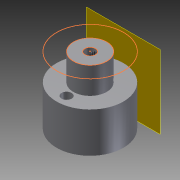
# Autodesk Inventor part: Jig_Bearing_Asm_Housing_Holder
Saved by Autodesk Inventor 2011 SP1 (Build 150282100, 282)
## iProperties
Created: 2011-04-25
Part Number: Jig_Bearing_Asm_Housing_Holder
Document SubType Name: Modeling
Designer: sungwook
Density: 1 g/cm^3
Author: sungwook
Autodesk Inventor part; units mm, degrees
ref_plane "YZ Plane" through (0, 0, 0) normal (1, 0, 0) x (0, 1, 0)
ref_plane "XY Plane" through (0, 0, 0) normal (0, 0, 1) x (1, 0, 0)
sketch "Sketch1" plane through (0, 0, 0) normal (0, 0, 1) x (1, 0, 0)
  circle A0 centre (0, 0) radius 5
  dimension "d0" = 10
  constraints: 1 centre point, 1 coincident
  measures "d0" diameter of A0
extrude "Extrusion1" add sketch "Sketch1" along normal blind 10
sketch "Sketch2" plane through (0, 0, 10) normal (0, 0, 1) x (1, 0, 0)
  circle A0 centre (0, 0) radius 5 projected
  circle A1 centre (0, 0) radius 0.8
  dimension "d3" = 1.6
  constraints: 1 centre point, 1 coincident
  measures "d3" diameter of A1
extrude "Extrusion2" cut sketch "Sketch2" against normal blind 2 contours A1
sketch "Sketch3" plane through (0, 0, 10) normal (0, 0, 1) x (1, 0, 0)
  circle A0 centre (0, 0) radius 0.8 projected
  circle A1 centre (0, 0) radius 5 projected
ref_plane "Work Plane1" through (0, 5, 0) normal (0, 1, 0) x (-1, 0, 0)
sketch "Sketch4" plane through (0, 5, 0) normal (0, 1, 0) x (-1, 0, 0)
  line L0 (-5, 0) -> (-5, 10) projected
  line L1 (5, 0) -> (5, 10) projected
  line L2 (0, -2) -> (0, 12) projected
  line L3 (-5, 10) -> (5, 10) projected
  point P0 (0, 0)
  point P1 (0, 9)
  dimension "d8" = 1
  constraints: 1 point on line
  measures "d8" distance from line of point (0, 9) L3
hole "Hole1" at (0, 5, 9) direction (0, -1, 0) diameter 1.181 depth 5 thread size "0-80 UNF" class "2B" standard "ANSI Unified Screw Threads"
sketch "Sketch5" plane through (0, 0, 10) normal (0, 0, 1) x (1, 0, 0)
  circle A0 centre (0, 0) radius 5 projected
  circle A1 centre (0, 0) radius 2.5
  circle A2 centre (0, 0) radius 5
  dimension "d16" = 5
  constraints: 2 centre point, 2 coincident, 1 concentric
  measures "d16" diameter of A1
extrude "Extrusion3" cut sketch "Sketch5" against normal blind 4
sketch "Sketch6" plane through (0, 0, 10) normal (0, 0, 1) x (1, 0, 0)
  circle A0 centre (0, 0) radius 2.5 projected
  circle A1 centre (0, 0) radius 0.8 projected
sketch "Sketch7" plane through (0, 0, 6) normal (0, 0, 1) x (1, 0, 0)
  circle A0 centre (0, 0) radius 2.5 projected
  circle A1 centre (0, -3.5) radius 0.75
  dimension "d19" = 1.5
  dimension "d20" = 3.5
  constraints: 1 centre point
  measures "d19" diameter of A1
  measures "d20" distance of A0.centre A1.centre
extrude "Extrusion4" cut sketch "Sketch7" against normal through all contours A1
body "Solid1"
